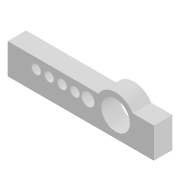
# Autodesk Inventor part: C_Unit_Cable_Holder_A
Saved by Autodesk Inventor 2020 (Build 240168000, 168)
## iProperties
Created: 2021-02-20
Part Number: C_Unit_Cable_Holder_A
Material: 一般
Document SubType Name: Modeling
Designer: ken113
Density: 1 g/cm^3
Appearance: 既定
Author: ken113
Autodesk Inventor part; units mm, degrees
ref_plane "YZ Plane" through (0, 0, 0) normal (1, 0, 0) x (0, 1, 0)
ref_plane "XZ Plane" through (0, 0, 0) normal (0, 1, 0) x (-1, 0, 0)
ref_plane "XY Plane" through (0, 0, 0) normal (0, 0, 1) x (1, 0, 0)
sketch "スケッチ1" plane through (0, 0, 0) normal (0, 0, 1) x (1, 0, 0)
  circle A0 centre (0, 11) radius 7.75
  line L0 (10.75, 0) -> (-48.5, 0)
  line L1 (-48.5, 0) -> (-48.5, 3.25)
  line L2 (-48.5, 3.25) -> (10.75, 3.25)
  line L3 (10.75, 3.25) -> (10.75, 0)
  circle A1 centre (0, 11) radius 10.75
  line L4 (10.75, 3.25) -> (10.75, 17.8822)
  circle A2 centre (-22, 11.0032) radius 2.5
  circle A3 centre (-29, 11.0065) radius 2.5
  circle A4 centre (-15, 11) radius 3.5
  circle A5 centre (-36, 11.0065) radius 2.5
  circle A6 centre (-43, 11.0065) radius 2.5
  circle A7 centre (-43, 11.0065) radius 5.5
  line L5 (-48.5, 3.25) -> (-48.5, 22.8758)
  line L6 (-51.01, 16.5065) -> (14.3021, 16.5065)
  point P0 (0, 0)
  point P1 (-9.2326, 16.5065)
  point P2 (-48.5, 16.5065)
  point P3 (10.75, 16.5065)
  point P4 (9.2326, 16.5065)
  dimension "d0" = 15.5
  dimension "d1" = 3
  dimension "d2" = 5
  dimension "d3" = 5
  dimension "d4" = 7
  dimension "d5" = 5
  dimension "d7" = 7
  dimension "d8" = 7
  dimension "d9" = 15
  dimension "d10" = 7
  dimension "d11" = 5
  dimension "d12" = 7
  dimension "d13" = 3
  dimension "d16" = 11
  constraints: 14 end point, 8 centre point, 6 tangent, 3 horizontal alignment, 2 parallel, 2 perpendicular, 1 horizontal, 1 vertical alignment
  measures "d0" diameter of A0
  measures "d1" radial gap between concentric circles of A0 A1
  measures "d2" diameter of A2
  measures "d3" diameter of A3
  measures "d4" diameter of A4
  measures "d5" diameter of A5
  measures "d7" distance of A2.centre A3.centre
  measures "d8" distance of A5.centre A3.centre
  measures "d9" distance of A0.centre A4.centre
  measures "d10" distance of A4.centre A2.centre
  measures "d11" diameter of A6
  measures "d12" distance of A6.centre A5.centre
  measures "d13" radial gap between concentric circles of A6 A7
  measures "d16" distance from line of A4.centre L0
extrude "押し出し1" add sketch "スケッチ1" along normal blind 10 contours A0 L6 A1 L2 | A0 L6 A1 | L2 A1 L6 A0 | L2 A1 | L6 L4 A1 | A1 L2 L3 L0 L1 | L2 L5 A7 A5 L6 A1 | A1 L4 L2 | A7 A5 | A7 L5 L6 picked at (-39.0972, 12.8262)
sketch "スケッチ3" plane through (0, 0, 10) normal (0, 0, 1) x (1, 0, 0)
  line L0 (-9.2326, 16.5065) -> (-48.5, 16.5065) projected
  line L1 (-48.5, 16.5065) -> (-48.5, 0) projected
  line L2 (-48.5, 0) -> (10.75, 0) projected
  line L3 (10.75, 0) -> (10.75, 16.5065) projected
  line L4 (10.75, 16.5065) -> (9.2326, 16.5065) projected
  arc A0 (9.2326, 16.5065) -> (-9.2326, 16.5065) centre (0, 11) ccw projected
  circle A1 centre (0, 11) radius 7.75 projected
  circle A2 centre (-43, 11.0065) radius 2.5 projected
  circle A3 centre (-15, 11) radius 3.5 projected
  circle A4 centre (-29, 11.0065) radius 2.5 projected
  circle A5 centre (-22, 11.0032) radius 2.5 projected
  circle A6 centre (-36, 11.0065) radius 2.5 projected
  line L5 (-48.5, 16.5065) -> (-48.5, 0) projected
  line L6 (-48.5, 0) -> (-58.5, 0)
  line L7 (-58.5, 0) -> (-58.5, 16.5065)
  line L8 (-58.5, 16.5065) -> (-48.5, 16.5065)
  line L9 (-48.5, 16.5065) -> (-48.5, 0)
  line L10 (10.75, 0) -> (20.75, 0)
  line L11 (20.75, 0) -> (20.75, 16.5065)
  line L12 (20.75, 16.5065) -> (10.75, 16.5065)
  line L13 (10.75, 16.5065) -> (10.75, 0)
  point P0 (0, 0)
  dimension "d17" = 10
  dimension "d18" = 10
  constraints: 16 end point, 4 parallel, 2 horizontal, 2 perpendicular, 1 coincident, 1 horizontal alignment
  measures "d17" distance of L7.end L8.end
  measures "d18" distance of L11.end L12.end
extrude "押し出し2" add sketch "スケッチ3" against normal up to surface (10 mm away) contours L1 L6 L7 L8 | L12 L11 L10 L3
